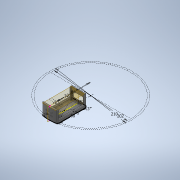
# Autodesk Inventor part: bat_mount003
Saved by Autodesk Inventor 2020 (Build 240168000, 168)
## iProperties
Created: 2024-02-10
Part Number: bat_mount003
Material: Типовые
Document SubType Name: Modeling
Designer: 4s
Density: 1 g/cm^3
Appearance: Гладкая — черная
Author: 4s
Autodesk Inventor part; units mm, degrees
ref_plane "YZ Plane" through (0, 0, 0) normal (1, 0, 0) x (0, 1, 0)
ref_plane "XZ Plane" through (0, 0, 0) normal (0, 1, 0) x (-1, 0, 0)
ref_plane "XY Plane" through (0, 0, 0) normal (0, 0, 1) x (1, 0, 0)
sketch "Эскиз1" plane through (0, 0, 0) normal (0, 1, 0) x (-1, 0, 0)
  circle A0 centre (0, 0) radius 101 construction
  line L0 (0, 0) -> (0, 101) construction
  line L1 (101, 0) -> (-101, 0) construction
  line L2 (19.5, 100.6566) -> (-17.5, 100.6566)
  line L3 (-17.5, 98.6566) -> (-17.5, 32.6566)
  line L4 (-15.5, 32.6566) -> (15.5, 32.6566)
  line L5 (17.5, 32.6566) -> (17.5, 98.6566)
  line L6 (17.5, 100.6566) -> (-17.5, 32.6566) construction
  line L7 (-17.5, 100.6566) -> (17.5, 32.6566) construction
  arc A1 (17.5, 98.6566) -> (15.5, 100.6566) centre (15.5, 98.6566) ccw
  arc A2 (15.5, 32.6566) -> (17.5, 34.6566) centre (15.5, 34.6566) ccw
  arc A3 (-17.5, 34.6566) -> (-15.5, 32.6566) centre (-15.5, 34.6566) ccw
  arc A4 (-15.5, 100.6566) -> (-17.5, 98.6566) centre (-15.5, 98.6566) ccw
  line L8 (16.5, 103.6566) -> (-16.5, 103.6566) construction
  line L9 (-19.5, 100.6566) -> (-19.5, 32.6566)
  line L10 (-16.5, 29.6566) -> (16.5, 29.6566)
  line L11 (19.5, 32.6566) -> (19.5, 100.6566)
  line L12 (19.5, 103.6566) -> (-19.5, 29.6566) construction
  line L13 (-19.5, 103.6566) -> (19.5, 29.6566) construction
  arc A5 (16.5, 29.6566) -> (19.5, 32.6566) centre (16.5, 32.6566) ccw
  arc A6 (-19.5, 32.6566) -> (-16.5, 29.6566) centre (-16.5, 32.6566) ccw
  arc A7 (-16.5, 103.6566) -> (-19.5, 100.6566) centre (-16.5, 100.6566) ccw
  arc A8 (19.5, 100.6566) -> (16.5, 103.6566) centre (16.5, 100.6566) ccw
  arc A9 (-16.9853, 103.6171) -> (16.9853, 103.6171) centre (0, 0) ccw construction
  arc A10 (16.9853, 103.6171) -> (-16.9853, 103.6171) centre (0, 0) ccw
  line L14 (-17.5, 100.6566) -> (-19.5, 100.6566)
  line L15 (-17.5, 32.6566) -> (-17.5, 29.8282)
  line L16 (17.5, 32.6566) -> (17.5, 29.8282)
  point P0 (0, 66.6566)
  dimension "d2" = 202
  dimension "d3" = 35
  dimension "d4" = 68
  dimension "d5" = 2
  dimension "d6" = 2
  dimension "d7" = 3
  dimension "d8" = 3
  dimension "d9" = 210
  constraints: 34 end point, 29 point on circle, 18 point on line, 17 tangent, 11 centre point, 6 equal radius, 5 midpoint, 4 horizontal, 4 parallel, 3 vertical, 2 coincident, 2 perpendicular, 1 other
  measures "d2" diameter of A0
  measures "d3" distance of L5.start L3.end
  measures "d4" distance of L3.end L2.end
  measures "d5" radius of A1
  measures "d6" distance between parallel lines of L3 L9
  measures "d7" distance between parallel lines of L10 L4
  measures "d8" radius of A5
  measures "d9" diameter of A9
extrude "Выдавливание3" add sketch "Эскиз1" against normal blind 1.5
ref_plane "РабПлоскость1" through (0, 28, 0) normal (0, 1, 0) x (1, 0, 0)
extrude "Выдавливание1" add sketch "Эскиз1" along normal up to surface (28 mm away) contours L2 L14 A7 A10 A8
ref_plane "РабПлоскость2" through (0, 7, 101.0346) normal (1, 0, 0) x (0, 0, -1)
sketch "Эскиз2" plane through (0, 7, 101.0346) normal (1, 0, 0) x (0, 0, -1)
  line L0 (-1, 0) -> (-1, 21) construction
  line L1 (-1, 21) -> (-2.9716, 21) construction
  line L2 (-2.9716, -9) -> (-2.9716, 21) construction
  line L3 (-2.5824, -8.5) -> (-2.5824, -8.5) construction
  line L4 (-2.5824, 21) -> (-2.5824, 21) construction
  line L5 (-2.5824, 21) -> (-2.5824, 21) construction
  line L6 (0.3781, -7) -> (68.3781, -7) projected
  line L7 (68.3781, -7) -> (71.3781, -7) projected
  line L8 (71.3781, -7) -> (68.3781, -7) projected
  line L9 (68.3781, -7) -> (0.3781, -7) projected
  line L10 (-2.5824, 21) -> (0.3781, 21) projected
  line L11 (0.3781, 21) -> (-2.5824, 21) projected
  line L12 (-2.5824, -8.5) -> (-2.5824, 21) projected
  line L13 (-2.5824, -8.5) -> (-2.5824, 21) projected
  point P0 (101.0346, -7)
extrude "Выдавливание4" add sketch "Эскиз1" along normal up to surface (28 mm away) contours A5 L10 A6 L15 L3 A3 L4 A2 L5 L16
sketch "Эскиз3" plane through (16.5, -1.5, 29.6566) normal (0, 0, -1) x (-1, 0, 0)
  line L0 (0, 0) -> (0, 29.5) construction
  line L1 (33, 0) -> (0, 0) construction
  line L2 (33, 0) -> (33, 29.5) construction
  line L3 (33, 29.5) -> (0, 29.5) construction
  line L4 (36, 29.5) -> (-3, 29.5) construction
  line L5 (-3, 1.5) -> (-3, 29.5) construction
  line L6 (36, 1.5) -> (-3, 1.5) construction
  line L7 (36, 1.5) -> (36, 29.5) construction
  line L8 (-3, 1.5) -> (-1, 1.5) construction
  line L9 (-3, 1.5) -> (-3, 0) construction
  line L10 (0, 0) -> (-3, 0) construction
  line L11 (0, 0) -> (0, 29.5) construction
  line L12 (0, 29.5) -> (-1, 29.5) construction
  line L13 (-1, 1.5) -> (-1, 29.5) construction
  line L14 (33.4853, 0) -> (33.4853, 29.5) construction
  line L15 (33, 0) -> (33, 29.5) construction
  line L16 (36, 0) -> (33, 0) construction
  line L17 (36, 1.5) -> (36, 0) construction
  line L18 (34, 1.5) -> (36, 1.5) construction
  line L19 (34, 1.5) -> (34, 29.5) construction
  line L20 (34, 29.5) -> (33, 29.5) construction
  line L21 (-0.4853, 0) -> (-0.4853, 29.5) construction
  line L22 (1, 29.5) -> (32, 29.5) construction
  line L23 (16.5, 29.5) -> (16.5, 1.5) construction
  line L24 (5.5, 6.5) -> (27.5, 6.5)
  line L25 (30.5, 9.5) -> (30.5, 18.5)
  line L26 (27.5, 21.5) -> (5.5, 21.5)
  line L27 (2.5, 18.5) -> (2.5, 9.5)
  line L28 (2.5, 6.5) -> (30.5, 21.5) construction
  line L29 (30.5, 6.5) -> (2.5, 21.5) construction
  arc A0 (5.5, 21.5) -> (2.5, 18.5) centre (5.5, 18.5) ccw
  arc A1 (30.5, 18.5) -> (27.5, 21.5) centre (27.5, 18.5) ccw
  arc A2 (27.5, 6.5) -> (30.5, 9.5) centre (27.5, 9.5) ccw
  arc A3 (2.5, 9.5) -> (5.5, 6.5) centre (5.5, 9.5) ccw
  point P0 (16.5, 14)
  dimension "d19" = 28
  dimension "d20" = 15
  dimension "d21" = 5
  dimension "d22" = 3
  constraints: 14 end point, 9 point on line, 8 point on circle, 8 tangent, 4 centre point, 3 equal radius, 3 midpoint, 2 parallel, 1 horizontal, 1 perpendicular, 1 vertical
  measures "d19" distance of L29.end L28.end
  measures "d20" distance of L28.end L29.start
  measures "d21" distance between parallel lines of L6 L24
  measures "d22" radius of A0
extrude "Выдавливание5" cut sketch "Эскиз3" against normal blind 10
sketch "Эскиз4" plane through (0, 28, 0) normal (0, 1, 0) x (1, 0, 0)
  line L0 (0, 0) -> (0, -84) construction
  line L1 (0, -84) -> (0, -89) construction
  line L2 (0, -89) -> (0, -84) construction
  line L3 (0, -84) -> (-17, -84) construction
  line L4 (-17, -84) -> (-17, -89) construction
  line L5 (-17, -89) -> (0, -89) construction
  line L6 (0, -84) -> (17, -84) construction
  line L7 (17, -89) -> (0, -89) construction
  line L8 (0, -84) -> (0, -32) construction
  dimension "d25" = 84
  dimension "d26" = 5
  dimension "d27" = 52
  constraints: 18 end point, 3 equal length, 2 point on line, 2 symmetric about line, 1 perpendicular, 1 vertical
  measures "d25" distance of L0.start L0.end
  measures "d26" distance of L0.end L1.end
  measures "d27" distance of L0.end L8.end
extrude "Выдавливание6" add sketch "Эскиз1" along normal blind 5 contours L11 A5 L16 L5 A1 L2 | A4 L3 L15 A6 L9 L14 L2
sketch "Эскиз5" plane through (-17.5, 0, 34.6566) normal (1, 0, 0) x (0, 0, -1)
  line L0 (2, 5) -> (2, 8) construction
  line L1 (5, 5) -> (2, 5) construction
  line L2 (5, 8) -> (5, 5) construction
  line L3 (5, 8) -> (2, 8) construction
  line L4 (2, 8) -> (2, 17) construction
  line L5 (5, 8) -> (2, 8) construction
  line L6 (5, 17) -> (5, 8) construction
  line L7 (5, 17) -> (2, 17) construction
  line L8 (2, 28) -> (0, 28) construction
  line L9 (0, 5) -> (0, 28) construction
  line L10 (0, 0) -> (0, 5) construction
  line L11 (2, 0) -> (0, 0) construction
  line L12 (2, 0) -> (2, 28) projected
  line L13 (0, 0) -> (0, 5) construction
  line L14 (-64, 5) -> (0, 5) construction
  line L15 (-64, 0) -> (-64, 5) construction
  line L16 (0, 0) -> (-64, 0) construction
  line L17 (-64, 0) -> (-66, 0) construction
  line L18 (-66, 0) -> (-64, 0) construction
  line L19 (-64, 0) -> (0, 0) construction
  line L20 (0, 0) -> (2, 0) projected
  line L21 (2, 0) -> (0, 0) construction
  line L22 (0, 0) -> (-64, 0) construction
  line L23 (0, 0) -> (2, 0) construction
  line L24 (2, 0) -> (2, 5) construction
  spline S0 degree 2 poles (0, 0) (2, 0) (2, 5) knots 1 1 1 2 2 2
  point P0 (34.6566, 0)
  point P1 (2, 4.9999)
  constraints: 2 collinear, 1 coincident, 3 other
extrude "Выдавливание7" add sketch "Эскиз5" along normal blind 35
ref_plane "РабПлоскость3" through (0, 28, 105) normal (0, 0, 1) x (1, 0, 0)
sketch "Эскиз6" plane through (0, 28, 105) normal (0, 0, 1) x (1, 0, 0)
  line L0 (-16.5, 0) -> (16.5, 0) construction
  line L1 (0, 0) -> (0, -28) construction
  circle A0 centre (0, -14) radius 9 construction
  line L2 (-1.5, -5) -> (1.5, -5)
  line L3 (1.5, -5) -> (1.5, -23)
  line L4 (1.5, -23) -> (-1.5, -23)
  line L5 (-1.5, -23) -> (-1.5, -5)
  line L6 (11, -23) -> (-11, -23) construction
  line L7 (-7.0442, -19.799) -> (-8.5442, -17.201)
  line L8 (-8.5442, -17.201) -> (7.0442, -8.201)
  line L9 (7.0442, -8.201) -> (8.5442, -10.799)
  line L10 (8.5442, -10.799) -> (-7.0442, -19.799)
  line L11 (8.5442, -17.201) -> (7.0442, -19.799)
  line L12 (7.0442, -19.799) -> (-8.5442, -10.799)
  line L13 (-8.5442, -10.799) -> (-7.0442, -8.201)
  line L14 (-7.0442, -8.201) -> (8.5442, -17.201)
  point P0 (0, -5)
  point P1 (0, -23)
  point P2 (-7.7942, -18.5)
  point P3 (7.7942, -9.5)
  point P4 (7.7942, -18.5)
  point P5 (-7.7942, -9.5)
  point P6 (3, -14)
  point P7 (1.5, -11.4019)
  point P8 (-1.5, -11.4019)
  point P9 (-3, -14)
  point P10 (-1.5, -16.5981)
  point P11 (1.5, -16.5981)
  dimension "d32" = 18
  dimension "d33" = 3
  dimension "d36" = 360
  constraints: 26 end point, 7 midpoint, 5 coincident, 2 parallel, 1 horizontal, 1 perpendicular, 1 point on line, 1 vertical, 1 vertical alignment, 37 other
  measures "d33" distance of L3.end L4.end
extrude "Выдавливание8" cut sketch "Эскиз6" against normal blind 0.5
ref_plane "РабПлоскость4" through (-15.5, 28, 32.6566) normal (0, 0, 1) x (1, 0, 0)
sketch "Эскиз7" plane through (-15.5, 28, 32.6566) normal (0, 0, 1) x (1, 0, 0)
  line L0 (-2, -28) -> (-2, -23)
  line L1 (-2, -28) -> (-2, -23)
  line L2 (-2, -28) -> (33, -28) construction
  line L3 (-2, -28) -> (0, -28)
  line L4 (0, -28) -> (31, -28) construction
  line L5 (31, -28) -> (33, -28) construction
  line L6 (33, -28) -> (33, -23) construction
  line L7 (33, -28) -> (33, -23) construction
  line L8 (0, -23.0001) -> (31, -23.0001) construction
  line L9 (31, -23.0001) -> (31, 0) construction
  line L10 (31, 0) -> (0, 0) construction
  line L11 (0, -23.0001) -> (0, 0) construction
  line L12 (29.5, -11) -> (29.5, -20) construction
  arc A0 (26.5, -23) -> (29.5, -20) centre (26.5, -20) ccw construction
  line L13 (26.5, -23) -> (4.5, -23) construction
  arc A1 (1.5, -20) -> (4.5, -23) centre (4.5, -20) ccw construction
  line L14 (1.5, -20) -> (1.5, -11) construction
  arc A2 (4.5, -8) -> (1.5, -11) centre (4.5, -11) ccw construction
  line L15 (4.5, -8) -> (26.5, -8) construction
  arc A3 (29.5, -11) -> (26.5, -8) centre (26.5, -11) ccw construction
  line L16 (-2, -28) -> (33, -28) construction
  line L17 (0, -23.0001) -> (31, -23.0001) construction
  line L18 (32, -29.5) -> (32, 0) construction
  line L19 (33, -28) -> (33, -23) construction
  line L20 (33, -23) -> (33, 0) construction
  line L21 (33, 0) -> (31, 0) construction
  line L22 (31, -23.0001) -> (31, 0) construction
  line L23 (0, -23.0001) -> (0, 0) construction
  line L24 (0, 0) -> (-2, 0) construction
  line L25 (-2, -23) -> (-2, 0) construction
  line L26 (-2, -28) -> (-2, -23)
  line L27 (-2, -28) -> (6, -28)
  line L28 (-2, -23) -> (-2, 0) construction
  line L29 (-2, -23) -> (1, -23.0001)
  line L30 (6, -28) -> (1, -28) construction
  line L31 (1, -28) -> (1, -23.0001) construction
  spline S0 degree 2 poles (6, -28) (1, -28) (1, -23.0001) knots 1 1 1 2 2 2
  line L32 (15.5, 6) -> (15.5, -36) construction
  line L33 (33, -28) -> (33, -23)
  line L34 (33, -28) -> (33, -23)
  line L35 (33, -28) -> (31, -28)
  line L36 (33, -28) -> (33, -23)
  line L37 (33, -28) -> (25, -28)
  line L38 (33, -23) -> (30, -23.0001)
  line L39 (25, -28) -> (30, -28) construction
  line L40 (30, -28) -> (30, -23.0001) construction
  spline S1 degree 2 poles (25, -28) (30, -28) (30, -23.0001) knots 1 1 1 2 2 2
  point P0 (15.5, -28)
  point P1 (35, -29.5)
  point P2 (31, -23.0001)
  point P3 (31, -23.0001)
  point P4 (31, -23.0001)
extrude "Выдавливание9" add sketch "Эскиз7" along normal up to surface (68 mm away)
